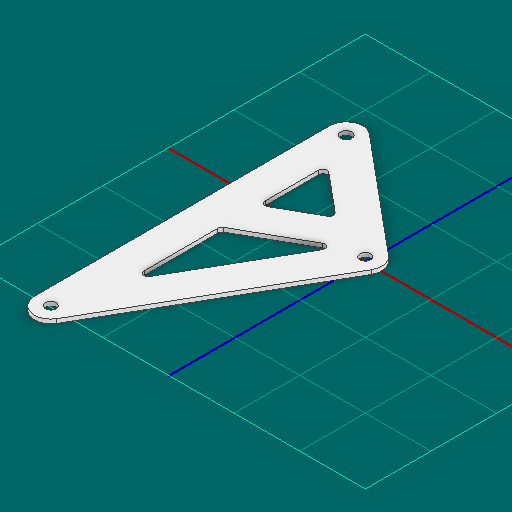
# Autodesk Inventor part: gusset
Saved by Autodesk Inventor 2025 (Build 290162000, 162)
## iProperties
Created: 2024-08-19
Part Number: gusset
Material: Acetal Resin, White
Document SubType Name: Modeling
Designer: averey
Density: 1.425 g/cm^3
Appearance: Smooth - White
Author: averey
Autodesk Inventor part; units mm, degrees
ref_plane "YZ Plane" through (0, 0, 0) normal (1, 0, 0) x (0, 1, 0)
ref_plane "XZ Plane" through (0, 0, 0) normal (0, 1, 0) x (-1, 0, 0)
ref_plane "XY Plane" through (0, 0, 0) normal (0, 0, 1) x (1, 0, 0)
sketch "main" plane through (0, 0, 0) normal (0, 0, 1) x (1, 0, 0)
  arc A0 (21.831, -6.1969) -> (19.4626, -4.8147) centre (20.2435, -6.1969) ccw
  line L0 (4.5808, -13.2233) -> (19.4626, -4.8147)
  circle A1 centre (-16.269, -6.907) radius 2.0955
  arc A2 (-21.7728, -3.7399) -> (-20.3351, -11.7845) centre (-16.269, -6.907) ccw
  line L1 (34.531, -43.9625) -> (34.531, 70.3375)
  arc A3 (-5.5129, -0.9469) -> (-3.356, -3.1208) centre (-4.137, -1.7387) ccw
  line L2 (-3.356, -3.1208) -> (21.0244, 10.6548)
  arc A4 (21.0244, 10.6548) -> (21.831, 12.037) centre (20.2435, 12.037) ccw
  line L3 (21.831, 12.037) -> (21.831, 40.6294)
  line L4 (18.8676, 41.4212) -> (-5.5129, -0.9469)
  line L5 (-21.7728, -3.7399) -> (22.6772, 73.5046)
  arc A5 (21.831, 40.6294) -> (18.8676, 41.4212) centre (20.2435, 40.6294) ccw
  circle A6 centre (28.181, 70.3375) radius 2.0955
  arc A7 (34.531, 70.3375) -> (22.6772, 73.5046) centre (28.181, 70.3375) ccw
  circle A8 centre (28.181, -43.9625) radius 2.1844
  arc A9 (24.1149, -48.84) -> (34.531, -43.9625) centre (28.181, -43.9625) ccw
  line L6 (24.1149, -48.84) -> (-20.3351, -11.7845)
  arc A10 (4.5808, -13.2233) -> (4.3452, -15.8248) centre (5.3617, -14.6055) ccw
  line L7 (21.831, -27.0116) -> (21.831, -6.1969)
  arc A11 (19.227, -28.2309) -> (21.831, -27.0116) centre (20.2435, -27.0116) ccw
  line L8 (4.3452, -15.8248) -> (19.227, -28.2309)
  point P0 (5.1171, -4.3382)
  point P1 (1.8899, -30.3122)
  point P2 (11.7861, -22.0279)
  dimension "d1" = 12.7
  dimension "d2" = 12.7
  dimension "d3" = 12.7
  dimension "d4" = 1.5875
  dimension "d5" = 12.7
  dimension "d6" = 1.5875
  dimension "d7" = 1.5875
  dimension "d10" = 114.3
  dimension "d12" = 12.7
  dimension "d13" = 12.7
  dimension "d14" = 13.187
  dimension "d16" = 44.45
  dimension "d17" = 12.7
  measures "d1" diameter of A2
  measures "d2" diameter of A7
  measures "d3" diameter of A9
  measures "d4" radius of A5
  measures "d5" distance between parallel lines of L2 L0
  measures "d6" radius of A3
  measures "d7" radius of A4
  measures "d10" distance of A8.centre A6.centre
  measures "d12" distance between parallel lines of L1 L7
  measures "d13" distance between parallel lines of L5 L4
  measures "d14" distance of A1.centre A3.centre
  measures "d16" horizontal distance of A8.centre A1.centre
  measures "d17" distance between parallel lines of L6 L8
sketch "Sketch1" plane through (0, 0, 0) normal (0, 1, 0) x (-1, 0, 0)
  arc A0 (38.1, 0.7102) -> (35.7316, 2.0923) centre (36.5125, 0.7102) ccw
  line L0 (20.8498, -6.3163) -> (35.7316, 2.0923)
  circle A1 centre (0, 0) radius 2.0955
  arc A2 (-5.5038, 3.1671) -> (-4.0661, -4.8775) centre (0, 0) ccw
  line L1 (50.8, -37.0554) -> (50.8, 77.2446)
  arc A3 (10.7561, 5.9602) -> (12.9129, 3.7863) centre (12.132, 5.1684) ccw
  line L2 (12.9129, 3.7863) -> (37.2934, 17.5619)
  arc A4 (37.2934, 17.5619) -> (38.1, 18.944) centre (36.5125, 18.944) ccw
  line L3 (38.1, 18.944) -> (38.1, 47.5364)
  line L4 (35.1366, 48.3282) -> (10.7561, 5.9602)
  line L5 (-5.5038, 3.1671) -> (38.9462, 80.4117)
  arc A5 (38.1, 47.5364) -> (35.1366, 48.3282) centre (36.5125, 47.5364) ccw
  circle A6 centre (44.45, 77.2446) radius 2.0955
  arc A7 (50.8, 77.2446) -> (38.9462, 80.4117) centre (44.45, 77.2446) ccw
  circle A8 centre (44.45, -37.0554) radius 2.1844
  arc A9 (40.3839, -41.9329) -> (50.8, -37.0554) centre (44.45, -37.0554) ccw
  line L6 (40.3839, -41.9329) -> (-4.0661, -4.8775)
  arc A10 (20.8498, -6.3163) -> (20.6142, -8.9178) centre (21.6307, -7.6984) ccw
  line L7 (38.1, -20.1045) -> (38.1, 0.7102)
  arc A11 (35.496, -21.3239) -> (38.1, -20.1045) centre (36.5125, -20.1045) ccw
  line L8 (20.6142, -8.9178) -> (35.496, -21.3239)
  constraints: 1 other
extrude "Extrusion1" add sketch "Sketch1" along normal blind 1.5875
body "Solid1"
